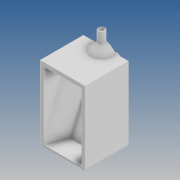
# Autodesk Inventor part: WaterDrainWell
Saved by Autodesk Inventor 2020 (Build 240168000, 168)
## iProperties
Created: 2019-08-07
Part Number: WaterDrainWell
Material: 일반
Document SubType Name: Modeling
Designer: Jeong Ji Hoon
Density: 1 g/cm^3
Appearance: 기본값
Author: Jeong Ji Hoon
## iProperties of the stored document _3D 인쇄.ipt
Created: 2019-08-07
Part Number: _3D 인쇄
Material: 일반
Document SubType Name: Modeling
Designer: Jeong Ji Hoon
Density: 1 g/cm^3
Appearance: 기본값
Author: Jeong Ji Hoon
Autodesk Inventor part; units mm, degrees
ref_plane "YZ Plane" through (0, 0, 0) normal (1, 0, 0) x (0, 1, 0)
ref_plane "XZ Plane" through (0, 0, 0) normal (0, 1, 0) x (-1, 0, 0)
ref_plane "XY Plane" through (0, 0, 0) normal (0, 0, 1) x (1, 0, 0)
sketch "스케치1" plane through (0, 0, 0) normal (0, 0, 1) x (1, 0, 0)
  line L0 (0, 0) -> (12, 0)
  line L1 (12, 0) -> (12, 20)
  line L2 (12, 20) -> (0, 20)
  line L3 (0, 20) -> (0, 0)
  dimension "d0" = 12
  dimension "d1" = 20
  constraints: 8 end point, 2 parallel, 1 horizontal, 1 perpendicular
  measures "d0" distance of L0.start L0.end
  measures "d1" distance of L0.end L1.end
extrude "돌출1" add sketch "스케치1" along normal blind 1.5
sketch "스케치2" plane through (0, 0, 1.5) normal (0, 0, 1) x (1, 0, 0)
  line L0 (0, 20) -> (0, 0) projected
  line L1 (0, 0) -> (12, 0) projected
  line L2 (12, 0) -> (12, 20) projected
  line L3 (12, 20) -> (0, 20) projected
  line L4 (1, 19) -> (1, 1)
  line L5 (1, 1) -> (11, 1)
  line L6 (11, 1) -> (11, 19)
  line L7 (11, 19) -> (1, 19)
  dimension "d4" = 1
  constraints: 8 end point, 3 other
  measures "d4" distance between parallel lines of L3 L7
extrude "돌출2" add sketch "스케치2" along normal blind 10
sketch "스케치3" plane through (1, 1, 1.5) normal (1, 0, 0) x (0, 0, -1)
  line L0 (0, 18) -> (0, 0) projected
  line L1 (0, 18) -> (-10, 18) projected
  line L2 (-10, 0) -> (-10, 18) projected
  line L3 (0, 0) -> (-10, 0) projected
  line L4 (-5, 0) -> (0, 13)
  line L5 (0, 16) -> (-8, 18)
  point P0 (1.5, -1)
  dimension "d7" = 13
  dimension "d8" = 5
  dimension "d9" = 2
  dimension "d10" = 2
  constraints: 4 end point, 3 point on line, 1 midpoint
  measures "d7" distance from line of L3 L4.end
  measures "d8" distance from line of L2 L4.start
  measures "d9" distance from line of L2 L5.end
  measures "d10" distance of L5.start L0.start
extrude "돌출3" add sketch "스케치3" along normal up to surface (10 mm away) contours L0 L5 L1 | L0 L3 L4
fillet "모깎기1" radius 1 3 edges at (0, 0, 5.75) (6, 0, 11.5) (12, 0, 5.75)
chamfer "모따기1" distance 5 distance2 2 1 edges at (1, 7.5, 4) measured on face at (1, 7.6795, 4.4667)
chamfer "모따기2" distance 5 distance2 2 1 edges at (11, 7.5, 4) measured on face at (11, 7.6795, 4.4667)
chamfer "모따기3" distance 2 angle 45 2 edges at (2.7846, 15.5, 1.5) (9.2154, 15.5, 1.5)
sketch "스케치4" plane through (1, 19, 9.5) normal (0, -0.9701425, 0.2425356) x (1, 0, 0)
  line L0 (6.4103, -8.2462) -> (3.5897, -8.2462) projected
  circle A0 centre (5, -7.8462) radius 0.6
  point P0 (-1, -13.8245)
  point P1 (5, -8.2462)
  point P2 (5.4472, -8.2462)
  point P3 (4.5528, -8.2462)
  dimension "d23" = 1.2
  dimension "d24" = 0.4
  constraints: 1 centre point, 1 midpoint, 1 vertical alignment
  measures "d23" diameter of A0
  measures "d24" distance of point (5, -8.246) A0.centre
extrude "돌출4" cut sketch "스케치4" against normal blind 10 contours L0 A0 picked at (5.0238, -7.9143)
sketch "스케치5" plane through (0, 20, 0) normal (0, 1, 0) x (1, 0, 0)
  ellipse E0 centre (6, -1.1623) end of major axis (6, -0.5438) minor radius 0.6 (5.5528, -0.75) -> (6.4472, -0.75) ccw projected
  circle A0 centre (6, -1.1623) radius 0.9
  circle A1 centre (6, -1.1623) radius 0.6083
  line L0 (6, -0.2623) -> (6, -2.0623) construction
  line L1 (6, -1.1623) -> (5.2628, -1.6785)
  line L2 (5.2628, -1.6785) -> (6, -2.0623)
  point P0 (5.5528, -1.5746)
  point P1 (6.4472, -1.5746)
  dimension "d27" = 1.8
  dimension "d30" = 0.2917
  dimension "d31" = 55
  constraints: 6 end point, 3 coincident, 3 point on circle, 1 centre point, 1 midpoint, 1 vertical, 4 other
  measures "d27" diameter of A0
  measures "d31" angle of L0 L1
extrude "돌출5" add sketch "스케치5" along normal blind 5 contours A1 E0 | A1 E0 | A0 L2 picked at (6.5993, -1.1125) picked at (6.0134, -1.7707) picked at (5.6788, -1.8253)
fillet "모깎기2" radius 0.2 1 edges at (6.4156, 25, 0.364)
chamfer "모따기4" distance 2 angle 45 2 edges at (5.6314, 20, 1.8704) (6.4156, 20, 0.364)
sketch "스케치6" plane through (0, 0, 0) normal (0, 0, -1) x (-1, 0, 0)
  line L0 (-1, 0) -> (-11, 0) projected
  line L1 (-6, 7.5) -> (-3.8349, 6.25)
  line L2 (-3.8349, 6.25) -> (-3.8349, 3.75)
  line L3 (-3.8349, 3.75) -> (-6, 2.5)
  line L4 (-6, 2.5) -> (-8.1651, 3.75)
  line L5 (-8.1651, 3.75) -> (-8.1651, 6.25)
  line L6 (-8.1651, 6.25) -> (-6, 7.5)
  line L7 (-6, 17.5) -> (-3.8349, 16.25)
  line L8 (-3.8349, 16.25) -> (-3.8349, 13.75)
  line L9 (-3.8349, 13.75) -> (-6, 12.5)
  line L10 (-6, 12.5) -> (-8.1651, 13.75)
  line L11 (-8.1651, 13.75) -> (-8.1651, 16.25)
  line L12 (-8.1651, 16.25) -> (-6, 17.5)
  point P0 (0, 0)
  point P1 (-6, 5)
  point P2 (-6, 0)
  point P3 (-6, 15)
  point P4 (-6, 0)
  dimension "d36" = 5
  dimension "d37" = 5
  dimension "d38" = 5
  dimension "d39" = 10
  constraints: 24 end point, 4 vertical alignment, 2 midpoint, 26 other
  measures "d36" distance from line of L0 point (-6, 5)
  measures "d37" distance of L1.start L3.end
  measures "d38" distance of L12.end L9.end
  measures "d39" distance of point (-6, 5) point (-6, 15)
extrude "돌출6" add sketch "스케치6" along normal blind 3
